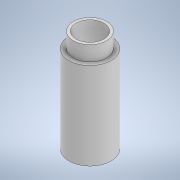
# Autodesk Inventor part: taoa
Saved by Autodesk Inventor 2022 (Build 260153000, 153)
## iProperties
Created: 2022-08-27
Part Number: taoa
Material: Generic
Document SubType Name: Modeling
Designer: alejo
Density: 1 g/cm^3
Appearance: Default
Author: alejo
Autodesk Inventor part; units mm, degrees
ref_plane "YZ Plane" through (0, 0, 0) normal (1, 0, 0) x (0, 1, 0)
ref_plane "XZ Plane" through (0, 0, 0) normal (0, 1, 0) x (-1, 0, 0)
ref_plane "XY Plane" through (0, 0, 0) normal (0, 0, 1) x (1, 0, 0)
sketch "Sketch1" plane through (0, 0, 0) normal (0, 1, 0) x (-1, 0, 0)
  circle A0 centre (0, 0) radius 140
  circle A1 centre (0, 0) radius 60
  dimension "d0" = 280
  dimension "d1" = 120
  constraints: 2 centre point, 2 coincident
  measures "d0" diameter of A0
  measures "d1" diameter of A1
extrude "Extrusion1" add sketch "Sketch1" along normal blind 30
sketch "Sketch3" plane through (0, 30, 0) normal (0, 1, 0) x (1, 0, 0)
  circle A0 centre (0, 0) radius 92.5
  circle A1 centre (0, 0) radius 140
  dimension "d12" = 185
  dimension "d18" = 280
  constraints: 2 centre point, 2 coincident
  measures "d12" diameter of A0
  measures "d18" diameter of A1
extrude "Extrusion3" add sketch "Sketch3" along normal blind 550
sketch "Sketch4" plane through (0, 580, 0) normal (0, 1, 0) x (1, 0, 0)
  circle A0 centre (0, 0) radius 60 projected
  circle A1 centre (0, 0) radius 111
  circle A2 centre (0, 0) radius 92.5
  dimension "d15" = 222
  dimension "d19" = 185
  constraints: 2 centre point, 2 coincident
  measures "d15" diameter of A1
  measures "d19" diameter of A2
extrude "Extrusion4" add sketch "Sketch4" along normal blind 100 contours A1
body "Solid1"
